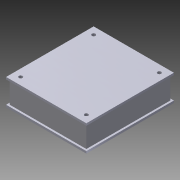
# Autodesk Inventor part: Part3
Saved by Autodesk Inventor 2015 (Build 190159000, 159)
## iProperties
Created: 2014-08-05
Part Number: Part3
Material: ABS Plastic
Document SubType Name: Modeling
Designer: Patrick Camilleri
Density: 1.06 g/cm^3
Appearance: Cool White
Author: Patrick Camilleri
Autodesk Inventor part; units mm, degrees
ref_plane "YZ Plane" through (0, 0, 0) normal (1, 0, 0) x (0, 1, 0)
ref_plane "XZ Plane" through (0, 0, 0) normal (0, 1, 0) x (-1, 0, 0)
ref_plane "XY Plane" through (0, 0, 0) normal (0, 0, 1) x (1, 0, 0)
sketch "Sketch1" plane through (0, 0, 0) normal (0, 0, 1) x (1, 0, 0)
  line L0 (-110, 120) -> (110, 120)
  line L1 (110, 120) -> (110, -120)
  line L2 (110, -120) -> (-110, -120)
  line L3 (-110, -120) -> (-110, 120)
  line L4 (-110, 120) -> (110, -120) construction
  line L5 (110, 120) -> (-110, -120) construction
  point P0 (0, 0)
  dimension "d0" = 220
  dimension "d1" = 240
  constraints: 12 end point, 2 midpoint, 2 parallel, 1 horizontal, 1 perpendicular
  measures "d0" distance of L1.end L2.end
  measures "d1" distance of L0.end L1.end
extrude "Extrusion1" add sketch "Sketch1" along normal blind 6
sketch "Sketch2" plane through (0, 0, 6) normal (0, 0, 1) x (1, 0, 0)
  line L0 (-110, -120) -> (-110, 120) projected
  line L1 (-110, -120) -> (110, -120) projected
  point P0 (0, 0)
  point P1 (-90, -100)
  dimension "d4" = 20
  dimension "d5" = 20
  measures "d4" distance from line of L0 point (-90, -100)
  measures "d5" distance from line of L1 point (-90, -100)
hole "Hole1" at (-90, -100, 6) direction (0, 0, -1) diameter 10 end through all
mirror "Mirror1" about plane through (0, 0, 0) normal (1, 0, 0) of "Hole1"
mirror "Mirror2" about plane through (0, 0, 0) normal (0, 1, 0) of "Hole1", "Mirror1"
sketch "Sketch4" plane through (0, 0, 6) normal (0, 0, 1) x (1, 0, 0)
  line L0 (110, 120) -> (-110, 120) projected
  line L1 (-110, 120) -> (-110, -120) projected
  line L2 (-105, 115) -> (105, 115)
  line L3 (105, 115) -> (105, -115)
  line L4 (105, -115) -> (-105, -115)
  line L5 (-105, -115) -> (-105, 115)
  line L6 (-105, 115) -> (105, -115) construction
  line L7 (105, 115) -> (-105, -115) construction
  line L8 (-102, 112) -> (102, 112)
  line L9 (102, 112) -> (102, -112)
  line L10 (102, -112) -> (-102, -112)
  line L11 (-102, -112) -> (-102, 112)
  point P0 (0, 0)
  dimension "d13" = 5
  dimension "d14" = 5
  dimension "d15" = 3
  constraints: 20 end point, 4 parallel, 2 midpoint, 2 perpendicular, 1 horizontal, 3 other
  measures "d13" distance between parallel lines of L0 L2
  measures "d14" distance between parallel lines of L1 L5
  measures "d15" distance between parallel lines of L5 L11
extrude "Extrusion2" add sketch "Sketch4" along normal blind 60
ref_plane "Work Plane1" through (0, 0, 36) normal (0, 0, 1) x (1, 0, 0)
mirror "Mirror3" about plane through (0, 0, 36) normal (0, 0, 1) of "Extrusion1"
sketch "Sketch5" plane through (-110, 120, 72) normal (0, 0, 1) x (1, 0, 0)
  line L0 (0, -240) -> (0, 0) projected
  line L1 (220, -240) -> (0, -240) projected
  point P0 (110, -120)
  point P1 (20, -220)
  dimension "d18" = 20
  dimension "d19" = 20
  measures "d18" distance from line of point (20, -220) L0
  measures "d19" distance from line of L1 point (20, -220)
hole "Hole2" at (-90, -100, 72) direction (0, 0, -1) diameter 10 end through all
mirror "Mirror4" about plane through (0, 0, 0) normal (1, 0, 0) of "Hole2"
mirror "Mirror5" about plane through (0, 0, 0) normal (0, 1, 0) of "Hole2", "Mirror4"
body "Solid1"
